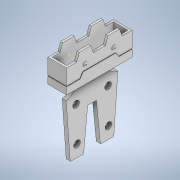
# Autodesk Inventor part: blade connector
Saved by Autodesk Inventor 2021 (Build 250183000, 183)
## iProperties
Created: 2021-03-29
Part Number: blade connector
Material: Generic
Document SubType Name: Modeling
Designer: newic
Density: 1 g/cm^3
Appearance: Default
Author: newic
Autodesk Inventor part; units mm, degrees
ref_plane "YZ Plane" through (0, 0, 0) normal (1, 0, 0) x (0, 1, 0)
ref_plane "XZ Plane" through (0, 0, 0) normal (0, 1, 0) x (-1, 0, 0)
ref_plane "XY Plane" through (0, 0, 0) normal (0, 0, 1) x (1, 0, 0)
sketch "Sketch1" plane through (0, 0, 0) normal (0, 1, 0) x (-1, 0, 0)
  line L0 (0, 0) -> (12.7, 0)
  line L1 (12.7, 0) -> (12.7, -57.15)
  line L2 (12.7, -57.15) -> (0, -57.15)
  line L3 (0, -57.15) -> (0, 0)
  line L4 (15.24, -59.69) -> (15.24, 2.54)
  line L5 (15.24, 2.54) -> (-2.54, 2.54)
  line L6 (-2.54, 2.54) -> (-2.54, -59.69)
  line L7 (-2.54, -59.69) -> (15.24, -59.69)
  dimension "d0" = 12.7
  dimension "d1" = 57.15
  dimension "d2" = 2.54
  constraints: 16 end point, 4 parallel, 2 perpendicular, 1 horizontal, 3 other
  measures "d0" distance of L1.end L2.end
  measures "d1" distance of L0.end L1.end
  measures "d2" distance between parallel lines of L1 L4
extrude "Extrusion1" add sketch "Sketch1" against normal blind 31.75
sketch "Sketch2" plane through (2.54, 0, 2.54) normal (1, 0, 0) x (0, 0, -1)
  point P0 (2.54, 0)
sketch "Sketch3" plane through (2.54, 0, 2.54) normal (1, 0, 0) x (0, 0, -1)
  line L0 (59.69, 0) -> (2.54, 0) projected
  line L1 (-1.2014, -9.525) -> (66.2927, -9.525)
  line L2 (31.115, 0) -> (31.115, -9.525)
  line L3 (0, 0) -> (0, -31.75) projected
  line L4 (0, -9.525) -> (8.255, -9.525)
  line L5 (62.23, 0) -> (62.23, -31.75) projected
  line L6 (62.23, -9.525) -> (53.975, -9.525)
  line L7 (31.115, -9.525) -> (34.925, -9.525)
  line L8 (31.115, -9.525) -> (27.305, -9.525)
  line L9 (0, -9.525) -> (9.525, -9.525)
  line L10 (31.115, -9.525) -> (25.4, -9.525)
  line L11 (31.115, -9.525) -> (36.83, -9.525)
  line L12 (62.23, -9.525) -> (52.705, -9.525)
  line L13 (0, 5.2281) -> (17.78, 5.2281)
  line L14 (17.78, 5.2281) -> (17.78, -9.525)
  line L15 (17.78, 0) -> (17.78, -2.54)
  line L16 (0, -2.54) -> (62.23, -2.54)
  line L17 (36.83, -9.525) -> (44.4179, 11.3227)
  line L18 (52.705, -9.525) -> (48.1245, 3.0598)
  line L19 (9.525, -9.525) -> (14.5428, 4.2614)
  line L20 (25.4, -9.525) -> (21.085, 2.3303)
  line L21 (36.83, -9.525) -> (52.705, -9.525)
  line L22 (-3.8276, -2.6318) -> (67.8028, -2.6318)
  line L23 (67.8028, -2.6318) -> (67.8028, 7.3948)
  line L24 (67.8028, 7.3948) -> (-3.8276, 7.3948)
  line L25 (-3.8276, 7.3948) -> (-3.8276, -2.6318)
  line L26 (-1.2014, -9.525) -> (-3.8276, -2.6318)
  line L27 (65.275, -9.525) -> (67.8028, -2.6318)
  point P0 (12.0339, -2.6318)
  point P1 (22.8911, -2.6318)
  point P2 (39.3389, -2.6318)
  point P3 (50.1961, -2.6318)
  dimension "d10" = 9.525
  dimension "d11" = 5.715
  dimension "d12" = 5.715
  dimension "d13" = 9.525
  dimension "d14" = 17.78
  dimension "d15" = 2.54
  dimension "d16" = 70
  dimension "d17" = 70
  dimension "d18" = 70
  dimension "d19" = 70
  constraints: 48 end point, 8 point on line, 3 horizontal, 2 parallel, 2 perpendicular, 2 vertical, 1 midpoint, 16 other
  measures "d10" distance of L4.start L9.end
  measures "d11" distance of L2.end L10.end
  measures "d12" distance of L2.end L11.end
  measures "d13" distance of L6.start L12.end
  measures "d14" distance of L13.start L13.end
  measures "d15" distance of L15.start L15.end
  measures "d16" angle to the sketch x axis of L19
  measures "d17" angle to the sketch x axis of L20
  measures "d18" angle to the sketch x axis of L17
  measures "d19" angle to the sketch x axis of L18
extrude "Extrusion2" cut sketch "Sketch3" against normal through all contours L18 L16 L17 L0 | L0 L17 L24 L23 L22 L5 L16 L18 | L17 L16 L2 L0 | L0 L19 L16 L3 L22 L25 L24 L17 | L18 L22 L17 L16 | L16 L5 L22 L18 | L2 L16 L20 L0 | L17 L22 L2 L16 | L22 L5 L1 L18 | L20 L16 L14 L0 | L2 L22 L20 L16 | L17 L1 L2 L22 | L22 L27 L1 L5 | L14 L16 L19 L0 | L20 L22 L14 L16 | L2 L1 L20 L22 | L22 L3 L1 L26 | L14 L22 L19 L16 | L22 L19 L1 L3 | L3 L16 L19 L22
sketch "Sketch4" plane through (2.54, -31.75, 2.54) normal (1, 0, 0) x (0, 0, -1)
  line L0 (0, 22.225) -> (0, 0) projected
  line L1 (0, 22.225) -> (0, 0)
  line L2 (0, 0) -> (0, 7.366)
  line L3 (0, 7.366) -> (62.23, 7.366)
  line L4 (62.23, 22.225) -> (62.23, 0) projected
  line L5 (12.0339, 29.1182) -> (22.8911, 29.1182) projected
  line L6 (17.4625, 29.1182) -> (17.4625, 4.5442)
  line L7 (50.1961, 29.1182) -> (39.3389, 29.1182) projected
  line L8 (44.7675, 29.1182) -> (44.7675, 5.1393)
  line L9 (17.4625, 7.366) -> (14.2875, 7.366)
  line L10 (44.7675, 7.366) -> (47.9425, 7.366)
  line L11 (47.9425, 7.366) -> (47.9425, 11.811)
  line L12 (14.2875, 7.366) -> (14.2875, 11.811)
  line L13 (17.4625, 11.811) -> (44.7675, 11.811)
  line L14 (0, 7.366) -> (0, 22.225)
  line L15 (0, 14.7955) -> (64.3687, 14.7955)
  line L16 (0, 16.7005) -> (64.3687, 16.7005)
  circle A0 centre (17.4625, 16.7005) radius 1.905
  circle A1 centre (44.7675, 16.7005) radius 1.905
  line L17 (46.6725, 11.811) -> (49.8475, 7.366)
  line L18 (15.5575, 11.811) -> (12.3825, 7.366)
  line L19 (15.5575, 11.811) -> (17.4625, 11.811)
  line L20 (46.6725, 11.811) -> (44.7675, 11.811)
  line L21 (12.8992, 6.9969) -> (15.8843, 11.176)
  line L22 (15.8843, 11.176) -> (17.4625, 11.176)
  line L23 (17.4625, 11.176) -> (44.7675, 11.176)
  line L24 (44.7675, 11.176) -> (46.3457, 11.176)
  line L25 (46.3457, 11.176) -> (49.3308, 6.9969)
  line L26 (0, 6.731) -> (62.23, 6.731)
  line L27 (12.8992, 6.9969) -> (12.7093, 6.731)
  line L28 (49.3308, 6.9969) -> (49.8475, 6.3495)
  point P0 (2.54, 31.75)
  point P1 (49.543, 6.731)
  point P2 (62.23, 6.731)
  point P3 (0, 7.366)
  point P4 (0, 6.731)
  dimension "d22" = 7.366
  dimension "d23" = 3.175
  dimension "d24" = 3.175
  dimension "d25" = 4.445
  dimension "d26" = 4.445
  dimension "d27" = 1.905
  dimension "d28" = 0.635
  dimension "d29" = 0.635
  constraints: 50 end point, 17 point on line, 4 perpendicular, 3 midpoint, 3 vertical, 2 centre point, 2 collinear, 2 parallel, 4 other
  measures "d22" distance of L0.end L2.end
  measures "d23" distance of L9.start L9.end
  measures "d24" distance of L10.start L10.end
  measures "d25" distance of L10.end L11.end
  measures "d26" distance of L9.end L12.end
  measures "d27" distance between parallel lines of L15 L16
  measures "d28" distance between parallel lines of L18 L21
  measures "d29" distance between parallel lines of L3 L26
sketch "Sketch5" plane through (-15.24, -31.75, -59.69) normal (-1, 0, 0) x (0, 0, 1)
  line L0 (0, 22.225) -> (0, 0)
  line L1 (0, 22.225) -> (0, 0)
  line L2 (0, 0) -> (0, 7.366)
  line L3 (0, 7.366) -> (62.23, 7.366)
  line L4 (62.23, 22.225) -> (62.23, 0)
  line L5 (12.0339, 29.1182) -> (22.8911, 29.1182)
  line L6 (17.4625, 29.1182) -> (17.4625, 4.5442)
  line L7 (50.1961, 29.1182) -> (39.3389, 29.1182)
  line L8 (44.7675, 29.1182) -> (44.7675, 5.1393)
  line L9 (17.4625, 7.366) -> (14.2875, 7.366)
  line L10 (44.7675, 7.366) -> (47.9425, 7.366)
  line L11 (47.9425, 7.366) -> (47.9425, 11.811)
  line L12 (14.2875, 7.366) -> (14.2875, 11.811)
  line L13 (17.4625, 11.811) -> (44.7675, 11.811)
  line L14 (0, 7.366) -> (0, 22.225)
  line L15 (0, 14.7955) -> (64.3687, 14.7955)
  line L16 (0, 16.7005) -> (64.3687, 16.7005)
  circle A0 centre (17.4625, 16.7005) radius 1.905
  circle A1 centre (44.7675, 16.7005) radius 1.905
  line L17 (46.6725, 11.811) -> (49.8475, 7.366)
  line L18 (15.5575, 11.811) -> (12.3825, 7.366)
  line L19 (15.5575, 11.811) -> (17.4625, 11.811)
  line L20 (46.6725, 11.811) -> (44.7675, 11.811)
  line L21 (12.8992, 6.9969) -> (15.8843, 11.176)
  line L22 (15.8843, 11.176) -> (17.4625, 11.176)
  line L23 (17.4625, 11.176) -> (44.7675, 11.176)
  line L24 (44.7675, 11.176) -> (46.3457, 11.176)
  line L25 (46.3457, 11.176) -> (49.3308, 6.9969)
  line L26 (0, 6.731) -> (62.23, 6.731)
  line L27 (12.8992, 6.9969) -> (12.7093, 6.731)
  line L28 (49.3308, 6.9969) -> (49.8475, 6.3495)
  point P0 (59.69, 31.75)
  point P1 (2.54, 31.75)
  point P2 (0, 6.731)
  point P3 (49.543, 6.731)
  point P4 (62.23, 6.731)
  point P5 (0, 7.366)
  dimension "d30" = 7.366
  dimension "d31" = 3.175
  dimension "d32" = 3.175
  dimension "d33" = 4.445
  dimension "d34" = 4.445
  dimension "d35" = 1.905
  dimension "d36" = 0.635
  dimension "d37" = 0.635
  constraints: 58 end point, 17 point on line, 4 perpendicular, 3 midpoint, 3 vertical, 2 centre point, 2 collinear, 2 parallel, 4 other
  measures "d30" distance of L0.end L14.start
  measures "d31" distance of L9.start L9.end
  measures "d32" distance of L10.start L10.end
  measures "d33" distance of L10.end L11.end
  measures "d34" distance of L9.end L12.end
  measures "d35" distance between parallel lines of L15 L16
  measures "d36" distance between parallel lines of L18 L21
  measures "d37" distance between parallel lines of L3 L26
extrude "Extrusion3" cut sketch "Sketch5" against normal blind 0.254 contours L3 L21 L27 L26 L0 | L18 L12 L21 L3 | L13 L8 L23 L6 | L6 L22 L21 L12 L18 L19 | L20 L17 L11 L25 L24 L8 | L4 L26 L28 L25 L3 | L17 L3 L25 L11
sketch "Sketch6" plane through (-15.24, -9.525, -34.29) normal (-1, 0, 0) x (0, 0, 1)
  line L0 (-25.4, 0) -> (-25.4, -22.225)
  line L1 (-25.4, 0) -> (-25.4, -22.225)
  line L2 (-25.4, -22.225) -> (-25.4, -14.859)
  line L3 (-25.4, -14.859) -> (36.83, -14.859)
  line L4 (36.83, 0) -> (36.83, -22.225)
  line L5 (-13.3661, 6.8933) -> (-2.5089, 6.8933)
  line L6 (-7.9375, 6.8933) -> (-7.9375, -17.6808)
  line L7 (24.7961, 6.8933) -> (13.9389, 6.8933)
  line L8 (19.3675, 6.8933) -> (19.3675, -17.0857)
  line L9 (-7.9375, -14.859) -> (-11.1125, -14.859)
  line L10 (19.3675, -14.859) -> (22.5425, -14.859)
  line L11 (22.5425, -14.859) -> (22.5425, -10.414)
  line L12 (-11.1125, -14.859) -> (-11.1125, -10.414)
  line L13 (-7.9375, -10.414) -> (19.3675, -10.414)
  line L14 (-25.4, -14.859) -> (-25.4, 0)
  line L15 (-25.4, -7.4295) -> (38.9686, -7.4295)
  line L16 (-25.4, -5.5245) -> (38.9686, -5.5245)
  circle A0 centre (-7.9375, -5.5245) radius 1.905
  circle A1 centre (19.3675, -5.5245) radius 1.905
  line L17 (21.2725, -10.414) -> (24.4475, -14.859)
  line L18 (-9.8425, -10.414) -> (-13.0175, -14.859)
  line L19 (-9.8425, -10.414) -> (-7.9375, -10.414)
  line L20 (21.2725, -10.414) -> (19.3675, -10.414)
  line L21 (-12.5008, -15.228) -> (-9.5157, -11.049)
  line L22 (-9.5157, -11.049) -> (-7.9375, -11.049)
  line L23 (-7.9375, -11.049) -> (19.3675, -11.049)
  line L24 (19.3675, -11.049) -> (20.9457, -11.049)
  line L25 (20.9457, -11.049) -> (23.9308, -15.228)
  line L26 (-25.4, -15.494) -> (36.83, -15.494)
  line L27 (-12.5008, -15.228) -> (-12.6907, -15.494)
  line L28 (23.9308, -15.228) -> (24.4475, -15.8755)
  point P0 (34.29, 9.525)
  point P1 (-22.86, 9.525)
  dimension "d40" = 7.366
  dimension "d41" = 3.175
  dimension "d42" = 3.175
  dimension "d43" = 4.445
  dimension "d44" = 4.445
  dimension "d45" = 1.905
  dimension "d46" = 0.635
  dimension "d47" = 0.635
  constraints: 58 end point, 17 point on line, 4 perpendicular, 3 midpoint, 3 vertical, 2 centre point, 2 collinear, 2 parallel, 4 other
  measures "d40" distance of L0.end L3.start
  measures "d41" distance of L9.start L9.end
  measures "d42" distance of L10.start L10.end
  measures "d43" distance of L10.end L11.end
  measures "d44" distance of L9.end L12.end
  measures "d45" distance between parallel lines of L15 L16
  measures "d46" distance between parallel lines of L18 L21
  measures "d47" distance between parallel lines of L3 L26
extrude "Extrusion4" cut sketch "Sketch4" against normal blind 0.254 contours L3 L21 L27 L26 L0 | L18 L12 L21 L3 | L13 L8 L23 L6 | L6 L22 L21 L12 L18 L19 | L20 L17 L11 L25 L24 L8 | L4 L26 L28 L25 L3 | L17 L3 L25 L11
sketch "Sketch7" plane through (2.54, -9.525, -22.86) normal (1, 0, 0) x (0, 0, -1)
  point P0 (-22.86, 9.525)
extrude "Extrusion5" add sketch "Sketch6" along normal blind 1.27 contours A0 L6 L16 | L16 L6 A0 | L6 L16 A0 | L6 A0 L16 | A1 L16 L8 | L8 L16 A1 | L16 A1 L8 | L8 A1 L16
sketch "Sketch8" plane through (2.54, -9.525, -22.86) normal (1, 0, 0) x (0, 0, -1)
  circle A0 centre (-7.9375, -5.5245) radius 1.905 projected
  circle A1 centre (-7.9375, -5.5245) radius 1.905
  circle A2 centre (19.3675, -5.5245) radius 1.905 projected
  circle A3 centre (19.3675, -5.5245) radius 1.905
  point P0 (-22.86, 9.525)
  constraints: 2 centre point, 2 coincident
extrude "Extrusion6" add sketch "Sketch8" along normal blind 1.27
sketch "Sketch9" plane through (-15.24, -9.525, -34.29) normal (-1, 0, 0) x (0, 0, 1)
  line L0 (-25.4, 0) -> (-25.4, -14.859) projected
  line L1 (-25.4, -15.494) -> (-12.713, -15.494) projected
  line L2 (-25.4, -14.859) -> (-25.146, -14.859)
  line L3 (-25.146, -14.859) -> (-25.146, -15.494)
  line L4 (-25.146, -15.494) -> (-25.4, -15.494)
  line L5 (-25.4, -15.494) -> (-25.4, -14.859)
  line L6 (24.4475, -14.859) -> (36.83, -14.859) projected
  line L7 (36.83, -15.494) -> (36.576, -15.494)
  line L8 (36.576, -15.494) -> (36.576, -14.859)
  line L9 (36.576, -14.859) -> (36.83, -14.859)
  line L10 (36.83, -14.859) -> (36.83, -15.494)
  point P0 (34.29, 9.525)
  dimension "d54" = 0.254
  dimension "d55" = 0.254
  constraints: 16 end point, 4 parallel, 2 horizontal, 2 perpendicular, 2 point on line
  measures "d54" distance of L3.end L4.end
  measures "d55" distance of L8.end L9.end
extrude "Extrusion7" cut sketch "Sketch9" against normal blind 2540
fillet "Fillet1" radius 1.27 4 edges at (-16.51, -15.0495, -44.1325) (-16.51, -15.0495, -16.8275) (3.81, -15.0495, -13.0175) (3.81, -15.0495, -40.3225)
sketch "Sketch10" plane through (-12.7, -31.75, 0) normal (1, 0, 0) x (0, 0, -1)
  line L0 (0, 0) -> (57.15, 0) projected
  line L1 (59.69, 6.731) -> (59.69, 0) projected
  line L2 (0, 0) -> (59.69, 0)
  line L3 (59.69, 0) -> (59.69, 2.54)
  line L4 (59.69, 2.54) -> (0, 2.54)
  line L5 (0, 2.54) -> (0, 0)
  point P0 (0, 31.75)
  dimension "d59" = 2.54
  constraints: 8 end point, 2 parallel, 1 horizontal, 1 perpendicular, 1 point on line
  measures "d59" distance of L3.end L2.end
extrude "Extrusion8" add sketch "Sketch10" along normal blind 13.97
sketch "Sketch11" plane through (0, -31.75, 0) normal (0, -1, 0) x (1, 0, 0)
  line L0 (-14.986, 2.286) -> (2.286, 2.286) projected
  line L1 (-15.24, -59.69) -> (2.54, -59.69) projected
  line L2 (2.54, -59.69) -> (2.54, 2.54) projected
  line L3 (2.54, 2.54) -> (-15.24, 2.54) projected
  line L4 (-15.24, 2.54) -> (-15.24, -59.69) projected
  line L5 (2.54, 2.54) -> (-15.24, 2.54) projected
  line L6 (-15.24, 2.54) -> (-15.24, -59.69) projected
  line L7 (2.54, 2.54) -> (-15.24, 2.54)
  line L8 (-6.35, 2.54) -> (-6.35, -73.2996)
  line L9 (-6.35, 2.54) -> (-4.445, 2.54)
  line L10 (-6.35, 2.54) -> (-8.255, 2.54)
  line L11 (-14.986, -59.436) -> (2.286, -59.436) projected
  line L12 (-8.255, 2.54) -> (-4.445, 2.54)
  line L13 (-4.445, 2.54) -> (-4.445, -59.436)
  line L14 (-4.445, -59.436) -> (-8.255, -59.436)
  line L15 (-8.255, -59.436) -> (-8.255, 2.54)
  point P0 (0, 0)
  point P1 (-8.255, 2.286)
  point P2 (-4.445, 2.286)
  dimension "d62" = 1.905
  dimension "d63" = 1.905
  constraints: 16 end point, 3 point on line, 2 parallel, 2 perpendicular, 1 horizontal, 1 midpoint, 1 vertical
  measures "d62" distance of L8.start L9.end
  measures "d63" distance of L8.start L10.end
extrude "Extrusion9" add sketch "Sketch11" along normal blind 76.2 contours L0 L8 L11 L15 | L0 L13 L11 L8
sketch "Sketch12" plane through (-4.445, -31.75, 2.286) normal (1, 0, 0) x (0, 0, -1)
  line L0 (-988.062, -700.5234) -> (-988.062, 1325.7378) construction
  line L1 (-988.062, 1325.7378) -> (444.4144, 1325.7378) construction
  line L2 (444.4144, 1325.7378) -> (444.4144, -700.5234) construction
  line L3 (444.4144, -700.5234) -> (-988.062, -700.5234) construction
  line L4 (0, 0) -> (61.722, 0) projected
  line L5 (0, 0) -> (0, -76.2) projected
  line L6 (61.722, -76.2) -> (0, -76.2) projected
  line L7 (61.722, 0) -> (61.722, -76.2) projected
  line L8 (0, 0) -> (61.722, 0) projected
  line L9 (0, 0) -> (6.35, 0)
  line L10 (6.35, 0) -> (6.35, -11.43)
  line L11 (-0.254, 0) -> (61.976, 0) projected
  line L12 (61.722, 0) -> (55.372, 0)
  line L13 (55.372, 0) -> (55.372, -11.43)
  line L14 (0, 0) -> (0, -63.5)
  line L15 (0, 0) -> (0, -76.2) projected
  line L16 (39.4357, -63.5) -> (61.722, -63.5)
  line L17 (61.722, 0) -> (61.722, -76.2) projected
  line L18 (0, -63.5) -> (10.16, -63.5)
  line L19 (61.722, -63.5) -> (51.562, -63.5)
  line L20 (10.16, -63.5) -> (22.2863, -63.5)
  line L21 (50.9718, -63.5) -> (38.862, -63.5)
  line L22 (50.5789, -63.5) -> (54.7064, -63.5)
  line L23 (54.7064, -63.5) -> (46.4514, -63.5)
  line L24 (30.861, 0) -> (30.861, -25.4)
  line L25 (6.35, -11.43) -> (10.1169, -62.9113)
  line L26 (22.918, -62.9292) -> (26.6755, -25.9708)
  line L27 (27.3072, -25.4) -> (34.4148, -25.4)
  line L28 (35.0465, -25.9708) -> (38.804, -62.9292)
  line L29 (51.6051, -62.9113) -> (55.372, -11.43)
  line L30 (6.35, 0) -> (16.51, 0)
  line L31 (55.372, 0) -> (45.212, 0)
  arc A0 (6.35, -11.43) -> (16.51, 0) centre (5.0802, -0.0708) ccw
  arc A1 (45.212, 0) -> (55.372, -11.43) centre (56.6418, -0.0708) ccw
  arc A2 (27.3072, -25.4) -> (26.6755, -25.9708) centre (27.3072, -26.035) ccw
  arc A3 (35.0465, -25.9708) -> (34.4148, -25.4) centre (34.4148, -26.035) ccw
  arc A4 (22.2863, -63.5) -> (22.918, -62.9292) centre (22.2863, -62.865) ccw
  arc A5 (10.1169, -62.9113) -> (10.7502, -63.5) centre (10.7502, -62.865) ccw
  arc A6 (38.804, -62.9292) -> (39.4357, -63.5) centre (39.4357, -62.865) ccw
  arc A7 (50.9718, -63.5) -> (51.6051, -62.9113) centre (50.9718, -62.865) ccw
  line L32 (16.51, -63.5) -> (16.51, -52.07)
  line L33 (46.4514, -63.5) -> (46.4514, -52.07)
  line L34 (30.861, -25.4) -> (30.861, -19.05)
  line L35 (30.861, -19.05) -> (15.621, -19.05)
  line L36 (30.861, -19.05) -> (46.101, -19.05)
  circle A8 centre (15.621, -19.05) radius 3.175
  circle A9 centre (46.101, -19.05) radius 3.175
  circle A10 centre (16.51, -52.07) radius 3.175
  circle A11 centre (46.4514, -52.07) radius 3.175
  point P0 (2.286, 31.75)
  point P1 (22.86, -63.5)
  point P2 (10.7502, -63.5)
  dimension "d107" = 6.35
  dimension "d110" = 11.43
  dimension "d113" = 6.35
  dimension "d114" = 11.43
  dimension "d115" = 63.5
  dimension "d116" = 10.16
  dimension "d117" = 10.16
  dimension "d118" = 12.7
  dimension "d119" = 12.7
  dimension "d120" = 4.1275
  dimension "d121" = 8.255
  dimension "d122" = 25.4
  dimension "d123" = 10.16
  dimension "d125" = 10.16
  dimension "d126" = 11.43
  dimension "d127" = 11.43
  dimension "d128" = 0.635
  dimension "d130" = 11.43
  dimension "d131" = 11.43
  dimension "d132" = 6.35
  dimension "d133" = 15.24
  dimension "d134" = 15.24
  dimension "d135" = 6.35
  dimension "d136" = 6.35
  dimension "d137" = 6.35
  dimension "d138" = 6.35
  constraints: 48 end point, 16 point on circle, 12 centre point, 11 point on line, 10 tangent, 5 equal radius, 4 coincident, 4 vertical, 3 perpendicular, 2 horizontal, 21 other
  measures "d107" distance of L4.start L9.end
  measures "d110" distance of L9.end L10.end
  measures "d113" distance of L4.end L12.end
  measures "d114" distance of L12.end L13.end
  measures "d115" distance of L4.start L14.end
  measures "d116" distance of L14.end L18.end
  measures "d117" distance of L19.start L19.end
  measures "d118" distance of L18.end point (22.86, -63.5)
  measures "d119" distance of L19.end L21.end
  measures "d120" distance of L22.start L22.end
  measures "d121" distance of L22.end L23.end
  measures "d122" distance of L24.start L24.end
  measures "d123" distance of L9.end L30.end
  measures "d125" distance of L12.end L31.end
  measures "d126" radius of A0
  measures "d127" radius of A1
  measures "d128" radius of A2
  measures "d130" distance of L32.start L32.end
  measures "d131" distance of L23.end L33.end
  measures "d132" distance of L24.end L34.end
  measures "d133" distance of L34.end L35.end
  measures "d134" distance of L34.end L36.end
  measures "d135" diameter of A8
  measures "d136" diameter of A9
  measures "d137" diameter of A10
  measures "d138" diameter of A11
extrude "Extrusion10" cut sketch "Sketch12" against normal blind 76.2 contours L4 L10 L25 A5 L20 L18 L5 | L4 A0 L10 | L18 L20 A4 L26 A2 L27 A3 L28 A6 L16 L7 L6 L5 | L4 L13 A1 | L16 A7 L29 L13 L4 L7 | A8 | A9 | A10 | A11
sketch "Sketch13" plane through (-15.24, -2.6318, -20.3511) normal (0, 1, 0) x (1, 0, 0)
  line L0 (15.24, -20.3511) -> (2.54, -20.3511) projected
  line L1 (2.54, 36.7989) -> (15.24, 36.7989) projected
  line L2 (2.54, -20.3511) -> (15.24, -20.3511)
  line L3 (15.24, -20.3511) -> (15.24, 36.7989)
  line L4 (15.24, 36.7989) -> (2.54, 36.7989)
  line L5 (2.54, 36.7989) -> (2.54, -20.3511)
  line L6 (15.748, 37.3069) -> (15.748, -20.8591)
  line L7 (15.748, -20.8591) -> (2.032, -20.8591)
  line L8 (2.032, -20.8591) -> (2.032, 37.3069)
  line L9 (2.032, 37.3069) -> (15.748, 37.3069)
  dimension "d141" = 0.508
  constraints: 16 end point, 4 parallel, 2 perpendicular, 1 horizontal, 3 other
  measures "d141" distance between parallel lines of L3 L6
extrude "Extrusion11" cut sketch "Sketch13" against normal blind 26.5684
body "Solid1"
